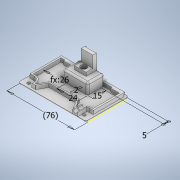
# Autodesk Inventor part: Deckel
Saved by Autodesk Inventor 2020.3 (Build 243373000, 373)
## iProperties
Created: 2020-09-26
Part Number: Deckel
Material: Generisch
Document SubType Name: Modeling
Designer: hpcwoess
Density: 1 g/cm^3
Appearance: Vorgabe
Author: hpcwoess
Autodesk Inventor part; units mm, degrees
ref_plane "YZ Plane" through (0, 0, 0) normal (1, 0, 0) x (0, 1, 0)
ref_plane "XY Plane" through (0, 0, 0) normal (0, 0, 1) x (1, 0, 0)
ref_plane "Arbeitsebene1" through (-34.5, -94, 30.7) normal (0, 1, 0) x (-1, 0, 0)
sketch "Skizze1" plane through (-34.5, -94, 30.7) normal (0, 1, 0) x (-1, 0, 0)
  circle A0 centre (-5, 5) radius 1.75 projected
  circle A1 centre (-67, 5) radius 1.75 projected
  arc A2 (-54.3246, 3.4866) -> (-54.0238, 3.1454) centre (-53.4437, 3.96) ccw projected
  line L0 (-54.3246, 3.4866) -> (-56.467, 7.4734) projected
  arc A3 (-56.467, 7.4734) -> (-57.3479, 8) centre (-57.3479, 7) ccw projected
  line L1 (-10, 8) -> (-14.6521, 8) projected
  arc A4 (-67, 0) -> (-65.2, 0.3352) centre (-67, 5) ccw projected
  line L2 (-67, 0) -> (-72, 0) projected
  line L3 (-72, 0) -> (-72, -34.5) projected
  line L4 (-62, -34.5) -> (-72, -34.5) projected
  line L5 (-62, -36) -> (-62, -34.5) projected
  line L6 (-62, -36) -> (-26, -36) projected
  line L7 (-26, -36) -> (-26, -34.5) projected
  line L8 (-9, -34.5) -> (-26, -34.5) projected
  line L9 (-9, -36) -> (-9, -34.5) projected
  line L10 (-9, -36) -> (-1, -36) projected
  arc A5 (-1, -36) -> (0, -35) centre (-1, -35) ccw projected
  line L11 (0, -35) -> (0, 0) projected
  line L12 (0, 0) -> (-5, 0) projected
  arc A6 (-10, 5) -> (-5, 0) centre (-5, 5) ccw projected
  line L13 (-10, 5) -> (-10, 8) projected
  arc A7 (-14.6521, 8) -> (-15.533, 7.4734) centre (-14.6521, 7) ccw projected
  line L14 (-15.533, 7.4734) -> (-20.4626, -1.7) projected
  line L15 (-24.2, -1.7) -> (-20.4626, -1.7) projected
  arc A8 (-24.2, -1.7) -> (-24.2487, -0.7) centre (-34.5, -1.7) ccw projected
  line L16 (-24.2487, -0.7) -> (-22.25, -0.7) projected
  line L17 (-22.25, 8) -> (-22.25, -0.7) projected
  line L18 (-22.25, 8) -> (-49.75, 8) projected
  line L19 (-49.75, -0.7) -> (-49.75, 8) projected
  line L20 (-49.75, -0.7) -> (-47, -0.7) projected
  line L21 (-47, -1.7) -> (-47, -0.7) projected
  line L22 (-50.4728, -1.7) -> (-47, -1.7) projected
  arc A9 (-50.4728, -1.7) -> (-54.0238, 3.1454) centre (-59.5709, -4.6437) ccw projected
  arc A10 (-74, -36) -> (-72, -38) centre (-72, -36) ccw projected
  line L23 (-74, -36) -> (-74, 8) projected
  arc A11 (-72, 10) -> (-74, 8) centre (-72, 8) ccw projected
  line L24 (-58.8, 10) -> (0, 10) projected
  arc A12 (2, 8) -> (0, 10) centre (0, 8) ccw projected
  line L25 (2, 8) -> (2, -36) projected
  arc A13 (0, -38) -> (2, -36) centre (0, -36) ccw projected
  line L26 (0, -38) -> (-72, -38) projected
  line L27 (-26.4, -35.6) -> (-61.6, -35.6)
  line L28 (-61.6, -35.6) -> (-61.6, -34.1)
  line L29 (-61.6, -34.1) -> (-71.6, -34.1)
  line L30 (-71.6, -34.1) -> (-71.6, -0.4)
  line L31 (-71.6, -0.4) -> (-67, -0.4)
  arc A14 (-67, -0.4) -> (-61.624, 4.4915) centre (-67, 5) ccw
  line L32 (-61.624, 4.4915) -> (-61.624, 7.6)
  line L33 (-61.624, 7.6) -> (-57.3479, 7.6)
  arc A15 (-56.8193, 7.284) -> (-57.3479, 7.6) centre (-57.3479, 7) ccw
  line L34 (-56.8193, 7.284) -> (-54.6769, 3.2973)
  arc A16 (-54.6769, 3.2973) -> (-54.2558, 2.8196) centre (-53.4437, 3.96) ccw
  arc A17 (-50.7686, -2.1) -> (-54.2558, 2.8196) centre (-59.5709, -4.6437) ccw
  line L35 (-50.7686, -2.1) -> (-46.6, -2.1)
  line L36 (-46.6, -2.1) -> (-46.6, -0.3)
  line L37 (-46.6, -0.3) -> (-49.35, -0.3)
  line L38 (-49.35, -0.3) -> (-49.35, 7.6)
  line L39 (-49.35, 7.6) -> (-22.65, 7.6)
  line L40 (-22.65, 7.6) -> (-22.65, -0.3)
  line L41 (-22.65, -0.3) -> (-24.6995, -0.3)
  arc A18 (-24.6081, -2.1) -> (-24.6995, -0.3) centre (-34.5, -1.7) ccw
  line L42 (-24.6081, -2.1) -> (-20.2235, -2.1)
  line L43 (-20.2235, -2.1) -> (-15.1807, 7.284)
  arc A19 (-14.6521, 7.6) -> (-15.1807, 7.284) centre (-14.6521, 7) ccw
  line L44 (-14.6521, 7.6) -> (-10.4, 7.6)
  line L45 (-10.4, 7.6) -> (-10.4, 5)
  arc A20 (-10.4, 5) -> (-5, -0.4) centre (-5, 5) ccw
  line L46 (-5, -0.4) -> (-0.4, -0.4)
  line L47 (-0.4, -0.4) -> (-0.4, -35)
  arc A21 (-1, -35.6) -> (-0.4, -35) centre (-1, -35) ccw
  line L48 (-1, -35.6) -> (-8.6, -35.6)
  line L49 (-8.6, -35.6) -> (-8.6, -34.1)
  line L50 (-8.6, -34.1) -> (-26.4, -34.1)
  line L51 (-26.4, -34.1) -> (-26.4, -35.6)
  line L52 (-59.6, -33.6) -> (-28.4, -33.6)
  line L53 (-28.4, -33.6) -> (-28.4, -32.1)
  line L54 (-28.4, -32.1) -> (-6.6, -32.1)
  line L55 (-6.6, -32.1) -> (-6.6, -33.6)
  line L56 (-6.6, -33.6) -> (-2.4, -33.6)
  line L57 (-2.4, -33.6) -> (-2.4, -2.4)
  line L58 (-2.4, -2.4) -> (-5, -2.4)
  arc A22 (-12.4, 5) -> (-5, -2.4) centre (-5, 5) ccw
  line L59 (-12.4, 5) -> (-12.4, 5.6)
  line L60 (-12.4, 5.6) -> (-13.8151, 5.6)
  line L61 (-13.8151, 5.6) -> (-19.0277, -4.1)
  line L62 (-19.0277, -4.1) -> (-26.9734, -4.1)
  arc A23 (-26.9734, -4.1) -> (-27.3691, 1.7) centre (-34.5, -1.7) ccw
  line L63 (-27.3691, 1.7) -> (-24.65, 1.7)
  line L64 (-24.65, 1.7) -> (-24.65, 5.6)
  line L65 (-24.65, 5.6) -> (-47.35, 5.6)
  line L66 (-47.35, 5.6) -> (-47.35, 1.7)
  line L67 (-47.35, 1.7) -> (-44.6, 1.7)
  line L68 (-44.6, 1.7) -> (-44.6, -4.1)
  line L69 (-44.6, -4.1) -> (-52.4291, -4.1)
  arc A24 (-52.4291, -4.1) -> (-55.416, 1.1905) centre (-59.5709, -4.6437) ccw
  arc A25 (-56.4387, 2.3505) -> (-55.416, 1.1905) centre (-53.4437, 3.96) ccw
  line L70 (-56.4387, 2.3505) -> (-58.1849, 5.6)
  line L71 (-58.1849, 5.6) -> (-59.624, 5.6)
  line L72 (-59.624, 5.6) -> (-59.624, 4.4046)
  arc A26 (-67, -2.4) -> (-59.624, 4.4046) centre (-67, 5) ccw
  line L73 (-67, -2.4) -> (-69.6, -2.4)
  line L74 (-69.6, -2.4) -> (-69.6, -32.1)
  line L75 (-69.6, -32.1) -> (-59.6, -32.1)
  line L76 (-59.6, -32.1) -> (-59.6, -33.6)
  line L77 (-65.2, 10) -> (-65.2, 0.3352) projected
  line L78 (-57.3479, 8) -> (-58.8, 8) projected
  line L79 (-58.8, 8) -> (-58.8, 10) projected
  line L80 (-72, 10) -> (-65.2, 10) projected
  line L81 (-58.8, 10) -> (-65.2, 10)
  line L82 (-58.8, 8) -> (-61.8, 8)
  line L83 (-61.8, 8) -> (-61.8, 4.5)
  point P0 (-34.5, -30.7)
  dimension "d0" = 0.4
  dimension "d1" = 2
  constraints: 106 end point, 26 point on circle, 13 centre point, 2 horizontal, 1 perpendicular, 57 other
  measures "d0" distance between parallel lines of L6 L27
  measures "d1" distance between parallel lines of L27 L52
extrude "Extrusion1" add sketch "Skizze1" against normal blind 2 contours L0 A3 L78 L79 L24 A12 L25 A13 L26 A10 L23 A11 L80 L77 A4 L2 L3 L4 L5 L6 L7 L8 L9 L10 A5 L11 L12 A6 L13 L1 A7 L14 L15 A8 L16 L17 L18 L19 L20 L21 L22 A9 A2 | A2 A9 L22 L21 L20 L19 L18 L17 L16 A8 L15 L14 A7 L1 L13 A6 L12 L11 A5 L10 L9 L8 L7 L6 L5 L4 L3 L2 A4 L77 L81 L79 L78 A3 L0 | L27 L28 L29 L30 L31 A14 L32 L33 A15 L34 A16 A17 L35 L36 L37 L38 L39 L40 L41 A18 L42 L43 A19 L44 L45 A20 L46 L47 A21 L48 L49 L50 L51 | L76 L75 L74 L73 A26 L72 L71 L70 A25 A24 L69 L68 L67 L66 L65 L64 L63 A23 L62 L61 L60 L59 A22 L58 L57 L56 L55 L54 L53 L52
sketch "Skizze4" plane through (-34.5, -94, 30.7) normal (0, 1, 0) x (-1, 0, 0)
  circle A0 centre (-5, 5) radius 1.75
  circle A1 centre (-67, 5) radius 1.75
  arc A2 (-54.3246, 3.4866) -> (-54.0238, 3.1454) centre (-53.4437, 3.96) ccw
  line L0 (-54.3246, 3.4866) -> (-56.467, 7.4734)
  arc A3 (-56.467, 7.4734) -> (-57.3479, 8) centre (-57.3479, 7) ccw
  line L1 (-57.3479, 8) -> (-62.024, 8)
  line L2 (-62.024, 8) -> (-62.024, 4.5108)
  arc A4 (-67, 0) -> (-62.024, 4.5108) centre (-67, 5) ccw
  line L3 (-67, 0) -> (-72, 0)
  line L4 (-72, 0) -> (-72, -34.5)
  line L5 (-62, -34.5) -> (-72, -34.5)
  line L6 (-62, -36) -> (-62, -34.5)
  line L7 (-62, -36) -> (-26, -36)
  line L8 (-26, -36) -> (-26, -34.5)
  line L9 (-9, -34.5) -> (-26, -34.5)
  line L10 (-9, -36) -> (-9, -34.5)
  line L11 (-9, -36) -> (-1, -36)
  arc A5 (-1, -36) -> (0, -35) centre (-1, -35) ccw
  line L12 (0, -35) -> (0, 0)
  line L13 (0, 0) -> (-5, 0)
  arc A6 (-10, 5) -> (-5, 0) centre (-5, 5) ccw
  line L14 (-10, 5) -> (-10, 8)
  line L15 (-10, 8) -> (-14.6521, 8)
  arc A7 (-14.6521, 8) -> (-15.533, 7.4734) centre (-14.6521, 7) ccw
  line L16 (-15.533, 7.4734) -> (-20.4626, -1.7)
  line L17 (-24.2, -1.7) -> (-20.4626, -1.7)
  arc A8 (-24.2, -1.7) -> (-24.2487, -0.7) centre (-34.5, -1.7) ccw
  line L18 (-24.2487, -0.7) -> (-22.25, -0.7)
  line L19 (-22.25, 8) -> (-22.25, -0.7)
  line L20 (-22.25, 8) -> (-49.75, 8)
  line L21 (-49.75, -0.7) -> (-49.75, 8)
  line L22 (-49.75, -0.7) -> (-47, -0.7)
  line L23 (-47, -1.7) -> (-47, -0.7)
  line L24 (-50.4728, -1.7) -> (-47, -1.7)
  arc A9 (-50.4728, -1.7) -> (-54.0238, 3.1454) centre (-59.5709, -4.6437) ccw
  arc A10 (-74, -36) -> (-72, -38) centre (-72, -36) ccw
  line L25 (-74, -36) -> (-74, 8)
  arc A11 (-72, 10) -> (-74, 8) centre (-72, 8) ccw
  line L26 (-72, 10) -> (0, 10)
  arc A12 (2, 8) -> (0, 10) centre (0, 8) ccw
  line L27 (2, 8) -> (2, -36)
  arc A13 (0, -38) -> (2, -36) centre (0, -36) ccw
  line L28 (0, -38) -> (-72, -38)
  line L29 (-26.4, -35.6) -> (-61.6, -35.6)
  line L30 (-61.6, -35.6) -> (-61.6, -34.1)
  line L31 (-61.6, -34.1) -> (-71.6, -34.1)
  line L32 (-71.6, -34.1) -> (-71.6, -0.4)
  line L33 (-71.6, -0.4) -> (-67, -0.4)
  arc A14 (-67, -0.4) -> (-61.624, 4.4915) centre (-67, 5) ccw
  line L34 (-61.624, 4.4915) -> (-61.624, 7.6)
  line L35 (-61.624, 7.6) -> (-57.3479, 7.6)
  arc A15 (-56.8193, 7.284) -> (-57.3479, 7.6) centre (-57.3479, 7) ccw
  line L36 (-56.8193, 7.284) -> (-54.6769, 3.2973)
  arc A16 (-54.6769, 3.2973) -> (-54.2558, 2.8196) centre (-53.4437, 3.96) ccw
  arc A17 (-50.7686, -2.1) -> (-54.2558, 2.8196) centre (-59.5709, -4.6437) ccw
  line L37 (-50.7686, -2.1) -> (-20.2235, -2.1)
  line L38 (-46.6, -0.3) -> (-49.35, -0.3)
  line L39 (-49.35, -0.3) -> (-49.35, 7.6)
  line L40 (-49.35, 7.6) -> (-22.65, 7.6)
  line L41 (-22.65, 7.6) -> (-22.65, -0.3)
  line L42 (-22.65, -0.3) -> (-24.6995, -0.3)
  line L43 (-24.6081, -2.1) -> (-20.2235, -2.1)
  line L44 (-20.2235, -2.1) -> (-15.1807, 7.284)
  arc A18 (-14.6521, 7.6) -> (-15.1807, 7.284) centre (-14.6521, 7) ccw
  line L45 (-14.6521, 7.6) -> (-10.4, 7.6)
  line L46 (-10.4, 7.6) -> (-10.4, 5)
  arc A19 (-10.4, 5) -> (-5, -0.4) centre (-5, 5) ccw
  line L47 (-5, -0.4) -> (-0.4, -0.4)
  line L48 (-0.4, -0.4) -> (-0.4, -35)
  arc A20 (-1, -35.6) -> (-0.4, -35) centre (-1, -35) ccw
  line L49 (-1, -35.6) -> (-8.6, -35.6)
  line L50 (-8.6, -35.6) -> (-8.6, -34.1)
  line L51 (-8.6, -34.1) -> (-26.4, -34.1)
  line L52 (-26.4, -34.1) -> (-26.4, -35.6)
  line L53 (-59.6, -33.6) -> (-28.4, -33.6)
  line L54 (-28.4, -33.6) -> (-28.4, -32.1)
  line L55 (-28.4, -32.1) -> (-6.6, -32.1)
  line L56 (-6.6, -32.1) -> (-6.6, -33.6)
  line L57 (-6.6, -33.6) -> (-2.4, -33.6)
  line L58 (-2.4, -33.6) -> (-2.4, -2.4)
  line L59 (-2.4, -2.4) -> (-5, -2.4)
  arc A21 (-12.4, 5) -> (-5, -2.4) centre (-5, 5) ccw
  line L60 (-12.4, 5) -> (-12.4, 5.6)
  line L61 (-12.4, 5.6) -> (-13.8151, 5.6)
  line L62 (-13.8151, 5.6) -> (-19.0277, -4.1)
  line L63 (-19.0277, -4.1) -> (-26.9734, -4.1)
  line L64 (-27.3691, 1.7) -> (-24.65, 1.7)
  line L65 (-24.65, 1.7) -> (-24.65, 5.6)
  line L66 (-24.65, 5.6) -> (-47.35, 5.6)
  line L67 (-47.35, 5.6) -> (-47.35, 1.7)
  line L68 (-47.35, 1.7) -> (-44.6, 1.7)
  line L69 (-19.0277, -4.1) -> (-52.4291, -4.1)
  arc A22 (-52.4291, -4.1) -> (-55.416, 1.1905) centre (-59.5709, -4.6437) ccw
  arc A23 (-56.4387, 2.3505) -> (-55.416, 1.1905) centre (-53.4437, 3.96) ccw
  line L70 (-56.4387, 2.3505) -> (-58.1849, 5.6)
  line L71 (-58.1849, 5.6) -> (-59.624, 5.6)
  line L72 (-59.624, 5.6) -> (-59.624, 4.4046)
  arc A24 (-67, -2.4) -> (-59.624, 4.4046) centre (-67, 5) ccw
  line L73 (-67, -2.4) -> (-69.6, -2.4)
  line L74 (-69.6, -2.4) -> (-69.6, -32.1)
  line L75 (-69.6, -32.1) -> (-59.6, -32.1)
  line L76 (-59.6, -32.1) -> (-59.6, -33.6)
  point P0 (-34.5, -30.7)
  point P1 (-34.5, -30.7)
  point P2 (-26.9734, -4.1)
  dimension "d4" = 0.4
  dimension "d5" = 2
  constraints: 154 end point, 46 point on circle, 25 centre point, 51 other
  measures "d4" distance between parallel lines of L7 L29
  measures "d5" distance between parallel lines of L29 L53
extrude "Extrusion2" add sketch "Skizze4" along normal blind 4 contours L29 L30 L31 L32 L33 A14 L34 L35 A15 L36 A16 A17 L37 L44 A18 L45 L46 A19 L47 L48 A20 L49 L50 L51 L52
sketch "Skizze5" plane through (-34.5, -96, 30.7) normal (0, -1, 0) x (1, 0, 0)
  line L0 (24, -18) -> (48, -18)
  line L1 (48, -18) -> (48, -33)
  line L2 (48, -33) -> (24, -33)
  line L3 (24, -33) -> (24, -18)
  line L4 (-2, 8) -> (-2, -36) projected
  line L5 (74, -36) -> (74, 8) projected
  line L6 (0, -38) -> (72, -38) projected
  line L7 (50, -16) -> (22, -16)
  line L8 (22, -16) -> (22, -35)
  line L9 (22, -35) -> (50, -35)
  line L10 (50, -35) -> (50, -16)
  point P0 (34.5, -30.7)
  dimension "d8" = 24
  dimension "d9" = 15
  dimension "d10" = 26
  dimension "d11" = 76
  dimension "d12" = 5
  dimension "d13" = 2
  constraints: 16 end point, 4 parallel, 2 perpendicular, 1 horizontal, 3 other
  measures "d8" distance of L0.start L0.end
  measures "d9" distance of L0.end L1.end
  measures "d10" distance between parallel lines of L4 L3
  measures "d11" distance between parallel lines of L5 L4
  measures "d12" distance between parallel lines of L2 L6
  measures "d13" distance between parallel lines of L0 L7
extrude "Extrusion3" add sketch "Skizze5" against normal blind 14 contours L0 L1 L2 L3 | L10 L9 L8 L7
extrude "Extrusion4" cut sketch "Skizze5" against normal blind 12 contours L0 L1 L2 L3
sketch "Skizze6" plane through (-34.5, -84, 30.7) normal (0, -1, 0) x (1, 0, 0)
  circle A0 centre (36, -25.5) radius 3.25
  line L0 (48, -18) -> (48, -33) projected
  line L1 (24, -18) -> (48, -18) projected
  line L2 (29.5, -21.75) -> (42.5, -21.75)
  line L3 (42.5, -21.75) -> (42.5, -29.25)
  line L4 (42.5, -29.25) -> (29.5, -29.25)
  line L5 (29.5, -29.25) -> (29.5, -21.75)
  line L6 (50, -35) -> (22, -35) projected
  line L7 (29.5, -29.25) -> (42.5, -29.25)
  line L8 (42.5, -29.25) -> (42.5, -35)
  line L9 (42.5, -35) -> (29.5, -35)
  line L10 (29.5, -35) -> (29.5, -29.25)
  point P0 (34.5, -30.7)
  dimension "d18" = 6.5
  dimension "d19" = 12
  dimension "d20" = 7.5
  dimension "d25" = 7.5
  dimension "d26" = 3.75
  dimension "d27" = 13
  dimension "d28" = 6.5
  constraints: 16 end point, 4 parallel, 2 horizontal, 2 perpendicular, 2 point on line, 1 centre point
  measures "d18" diameter of A0
  measures "d19" distance from line of A0.centre L0
  measures "d20" distance from line of L1 A0.centre
  measures "d25" distance between parallel lines of L2 L4
  measures "d26" distance from line of L4 A0.centre
  measures "d27" distance of L2.start L2.end
  measures "d28" distance from line of L3 A0.centre
sketch "Skizze7" plane through (37.1, -94, -3.4) normal (1, 0, 0) x (0, 0, -1)
  line L0 (1.5, 4) -> (0.9, 4) projected
  line L1 (3.9, 0) -> (3.9, -2) projected
  line L2 (1.5, 4) -> (3.9, 4)
  line L3 (3.9, 4) -> (3.9, 0)
  line L4 (3.9, 0) -> (1.5, 0)
  line L5 (1.5, 0) -> (1.5, 4)
  line L6 (3.9, 0) -> (2.2, 0)
  line L7 (2.2, 0) -> (2.2, 2.2)
  line L8 (2.2, 2.2) -> (3.9, 2.2)
  line L9 (3.9, 2.2) -> (3.9, 0)
  line L10 (0, 0) -> (0, 4) projected
  line L11 (1.5, 4) -> (0, 4)
  line L12 (0, 4) -> (0, 0)
  line L13 (0, 0) -> (1.5, 0)
  line L14 (1.5, 0) -> (1.5, 4)
  point P0 (-3.4, 94)
  point P1 (2.2, 0)
  point P2 (3.9, 2.2)
  point P3 (1.5, 0)
  dimension "d21" = 1.7
  dimension "d22" = 2.2
  constraints: 24 end point, 6 parallel, 3 horizontal, 3 perpendicular
  measures "d21" distance of L7.end L8.end
  measures "d22" distance of L6.end L7.end
extrude "Extrusion5" add sketch "Skizze7" against normal up to surface (71.2 mm away) contours L5 L13 L10 L11 L0 | L2 L3 L8 L7 L4 L5
sketch "Skizze8" plane through (-34.5, -96, 30.7) normal (0, -1, 0) x (1, 0, 0)
  point P0 (34.5, -30.7)
extrude "Extrusion6" add sketch "Skizze6" against normal blind 6 contours L2 L3 L4 L5
sketch "Skizze9" plane through (-34.5, -84, 30.7) normal (0, -1, 0) x (1, 0, 0)
  circle A0 centre (36, -25.5) radius 3.25
  line L0 (48, -18) -> (48, -33)
  line L1 (24, -18) -> (48, -18)
  line L2 (29.5, -21.75) -> (42.5, -21.75)
  line L3 (42.5, -21.75) -> (42.5, -29.25)
  line L4 (42.5, -29.25) -> (29.5, -29.25)
  line L5 (29.5, -29.25) -> (29.5, -21.75)
  line L6 (50, -35) -> (22, -35)
  line L7 (29.5, -29.25) -> (42.5, -29.25)
  line L8 (42.5, -29.25) -> (42.5, -35)
  line L9 (42.5, -35) -> (29.5, -35)
  line L10 (29.5, -35) -> (29.5, -29.25)
  point P0 (34.5, -30.7)
  point P1 (34.5, -30.7)
  dimension "d31" = 6.5
  dimension "d32" = 12
  dimension "d33" = 7.5
  dimension "d34" = 7.5
  dimension "d35" = 3.75
  dimension "d36" = 13
  dimension "d37" = 6.5
  constraints: 22 end point, 4 parallel, 2 horizontal, 2 perpendicular, 2 point on line, 1 centre point
  measures "d31" diameter of A0
  measures "d32" distance from line of A0.centre L0
  measures "d33" distance from line of L1 A0.centre
  measures "d34" distance between parallel lines of L2 L4
  measures "d35" distance from line of L4 A0.centre
  measures "d36" distance of L2.start L2.end
  measures "d37" distance from line of L3 A0.centre
extrude "Extrusion7" add sketch "Skizze9" against normal blind 19 contours L4 L8 L6 L10
sketch "Skizze10" plane through (-34.5, -78, 30.7) normal (0, 1, 0) x (1, 0, 0)
  line L0 (29.5, 21.75) -> (42.5, 21.75) projected
  line L1 (42.5, 21.75) -> (42.5, 29.25) projected
  line L2 (42.5, 29.25) -> (29.5, 29.25) projected
  line L3 (29.5, 29.25) -> (29.5, 21.75) projected
  circle A0 centre (36, 25.5) radius 3.25 projected
  point P0 (34.5, 30.7)
extrude "Extrusion8" cut sketch "Skizze10" against normal blind 10 contours A0
fillet "Rundung1" radius 2 20 edges at (1.5, -96, 12.7) (13.5, -96, 5.2) (1.5, -96, -2.3) (-10.5, -96, 5.2) (1.5, -82, 14.7) (15.5, -82, 5.2) (1.5, -84, -2.3) (-10.5, -84, 5.2) (1.5, -84, 12.7) (13.5, -84, 5.2) (-12.5, -82, 5.2) (15.5, -88, 14.7) (-12.5, -88, 14.7) (1.5, -65, -4.3) (8, -73.5, -4.3) (-5, -73.5, -4.3) (11.75, -82, -4.3) (-8.75, -82, -4.3) (15.5, -86, -4.3) (-12.5, -86, -4.3)
fillet "Rundung2" radius 2 7 edges at (-35.9142, -96, 40.1142) (-36.5, -96, 16.7) (-35.9142, -96, -6.7142) (1.5, -96, -7.3) (38.9142, -96, -6.7142) (39.5, -96, 16.7) (38.9142, -96, 40.1142)
sketch "Skizze11" plane through (-34.5, -84, 30.7) normal (0, -1, 0) x (1, 0, 0)
  line L0 (27.3428, -21.9377) -> (49.5374, -21.9377) construction
  line L1 (49.5374, -21.9377) -> (49.5374, -30.3697) construction
  line L2 (49.5374, -30.3697) -> (27.3428, -30.3697) construction
  line L3 (27.3428, -30.3697) -> (27.3428, -21.9377) construction
  line L4 (30.4911, -29.0852) -> (27.7796, -29.0852)
  line L5 (27.7796, -29.0852) -> (27.7796, -28.3705)
  line L6 (27.7796, -28.3705) -> (28.6702, -28.3705)
  line L7 (28.6702, -28.3705) -> (28.6702, -22.8)
  line L8 (28.6702, -22.8) -> (27.7796, -22.8)
  line L9 (27.7796, -22.8) -> (27.7796, -22.0852)
  line L10 (27.7796, -22.0852) -> (30.4911, -22.0852)
  line L11 (30.4911, -22.0852) -> (30.4911, -22.8)
  line L12 (30.4911, -22.8) -> (29.6005, -22.8)
  line L13 (29.6005, -22.8) -> (29.6005, -28.3705)
  line L14 (29.6005, -28.3705) -> (30.4911, -28.3705)
  line L15 (30.4911, -28.3705) -> (30.4911, -29.0852)
  spline S0 degree 2 poles (45.6143, -22.8851) (46.0114, -23.3502) (46.4538, -24.7116) (46.4538, -25.5852) knots 0 0 0 1 2 2 2
  spline S1 degree 2 poles (46.4538, -25.5852) (46.4538, -26.4361) (46.0227, -27.8145) (45.6143, -28.2797) knots 0 0 0 1 2 2 2
  spline S2 degree 2 poles (45.6143, -28.2797) (45.1832, -28.7675) (44.043, -29.2327) (43.3566, -29.2327) knots 0 0 0 1 2 2 2
  spline S3 degree 2 poles (43.3566, -29.2327) (42.6475, -29.2327) (41.513, -28.7505) (41.0989, -28.2797) knots 0 0 0 1 2 2 2
  spline S4 degree 2 poles (41.0989, -28.2797) (40.6961, -27.8145) (40.265, -26.4474) (40.265, -25.5852) knots 0 0 0 1 2 2 2
  spline S5 degree 2 poles (40.265, -25.5852) (40.265, -24.706) (40.7018, -23.3672) (41.1046, -22.8851) knots 0 0 0 1 2 2 2
  spline S6 degree 2 poles (41.1046, -22.8851) (41.513, -22.4199) (42.6532, -21.9377) (43.3566, -21.9377) knots 0 0 0 1 2 2 2
  spline S7 degree 2 poles (43.3566, -21.9377) (44.0714, -21.9377) (45.2172, -22.4369) (45.6143, -22.8851) knots 0 0 0 1 2 2 2
  spline S8 degree 2 poles (45.4838, -25.5852) (45.4838, -24.8932) (45.1832, -23.821) (44.9109, -23.4693) knots 0 0 0 1 2 2 2
  spline S9 degree 2 poles (44.9109, -23.4693) (44.6329, -23.1063) (43.8501, -22.7432) (43.3623, -22.7432) knots 0 0 0 1 2 2 2
  spline S10 degree 2 poles (43.3623, -22.7432) (42.8574, -22.7432) (42.0973, -23.0949) (41.808, -23.4693) knots 0 0 0 1 2 2 2
  spline S11 degree 2 poles (41.808, -23.4693) (41.53, -23.8267) (41.235, -24.9045) (41.235, -25.5852) knots 0 0 0 1 2 2 2
  spline S12 degree 2 poles (41.235, -25.5852) (41.235, -26.9637) (42.3923, -28.4272) (43.3623, -28.4272) knots 0 0 0 1 2 2 2
  spline S13 degree 2 poles (43.3623, -28.4272) (44.3323, -28.4272) (45.4838, -26.9637) (45.4838, -25.5852) knots 0 0 0 1 2 2 2
  point P0 (34.5, -30.7)
  constraints: 2 other
extrude "Extrusion9" cut sketch "Skizze11" against normal mid plane 1
chamfer "Fase1" distance 0.5 distance2 4 1 edges at (0.9961, -90, 28.6) measured on face at (0.9961, -90, 28.1)
chamfer "Fase2" distance 0.5 distance2 4 6 edges at (16.2005, -90, 28.351) (17.5959, -90, 31.3549) (19.9939, -90, 33.7342) (21.2481, -90, 35.9906) (22.54, -90, 38.215) (24.9859, -90, 38.3) measured on face at (16.6845, -90, 28.2257) measured on face at (21.6886, -90, 35.754) measured on face at (24.9859, -90, 37.8) measured on face at (18.0038, -90, 31.0658) measured on face at (22.7965, -90, 37.7858) measured on face at (20.369, -90, 33.4035)
chamfer "Fase3" distance 0.5 distance2 4 2 edges at (28.8658, -90, 31.7059) (34.8, -90, 30.3)
chamfer "Fase4" distance 0.5 distance2 4 1 edges at (27.124, -90, 35.5347) measured on face at (26.624, -90, 35.5347)
chamfer "Fase5" distance 0.5 distance2 4 3 edges at (-16.6636, -90, 33.0421) (-19.54, -90, 38.215) (-21.9739, -90, 38.3) measured on face at (-19.7965, -90, 37.7858) measured on face at (-21.9739, -90, 37.8) measured on face at (-17.104, -90, 32.8054)
chamfer "Fase6" distance 0.5 distance2 4 3 edges at (-25.6816, -90, 31.8816) (-24.1, -90, 36.75) (-31.8, -90, 30.3) measured on face at (-25.3281, -90, 31.5281) measured on face at (-23.6, -90, 36.75) measured on face at (-31.8, -90, 29.8)
sketch "Skizze12" plane through (-34.5, -94, 30.7) normal (0, 1, 0) x (1, 0, 0)
  line L0 (0, -10) -> (59, -10) projected
  line L1 (65, -10) -> (59, -10)
  line L2 (59, -10) -> (59, 0)
  line L3 (59, 0) -> (65, 0)
  line L4 (65, 0) -> (65, -10)
  circle A0 centre (67, -5) radius 1.75 projected
  point P0 (34.5, 30.7)
  point P1 (72, -10)
  dimension "d66" = 6
  dimension "d67" = 10
  dimension "d68" = 2
  constraints: 8 end point, 2 parallel, 1 horizontal, 1 perpendicular, 1 point on line
  measures "d66" distance of L2.end L3.end
  measures "d67" distance of L0.end L2.end
  measures "d68" distance from line of A0.centre L4
extrude "Extrusion10" add sketch "Skizze12" along normal blind 4 contours L1 L2 L3 L4
sketch "Skizze13" plane through (-34.5, -90, 30.7) normal (0, 1, 0) x (1, 0, 0)
  line L0 (65, -10) -> (65, 0) projected
  line L1 (59, -7.1) -> (59, -5.6) projected
  line L2 (59, -10) -> (65, -10) projected
  line L3 (62, -10) -> (62, 0)
  line L4 (65, 0) -> (63.8679, 0) projected
  line L5 (60, 0) -> (60, -10)
  line L6 (64, 0) -> (64, -10)
  line L7 (60, -4.5) -> (60.1, -4.5)
  line L8 (60.1, -4.5) -> (60.1, -5.5)
  line L9 (60.1, -5.5) -> (60, -5.5)
  line L10 (60, -5.5) -> (60, -4.5)
  line L11 (60, 0) -> (62, 0)
  line L12 (61.5447, 0) -> (59, 0) projected
  line L13 (60, -10) -> (62, -10)
  line L14 (60, 0) -> (62, 0)
  line L15 (62, 0) -> (62, 3.925)
  line L16 (62, 3.925) -> (60, 3.925)
  line L17 (60, 3.925) -> (60, 0)
  point P0 (34.5, 30.7)
  point P1 (62, 0)
  dimension "d72" = 2
  dimension "d73" = 2
  dimension "d74" = 0.1
  dimension "d75" = 1
  dimension "d76" = 4.5
  constraints: 26 end point, 4 parallel, 4 point on line, 3 perpendicular, 2 collinear, 2 horizontal, 2 vertical, 1 midpoint
  measures "d72" distance between parallel lines of L5 L3
  measures "d73" distance between parallel lines of L6 L3
  measures "d74" distance of L8.end L9.end
  measures "d75" distance of L7.end L8.end
  measures "d76" distance from line of L8.end L2
revolve "Umdrehung1" cut sketch "Skizze13" angle 360 about axis through (27.5, -90, 40.7) along (0, 0, -1) contours L5 L9 L8 L7 L11 L3 L2 | L11 L17 L16 L15
sketch "Skizze14" plane through (37.1, -94, -5.6) normal (1, 0, 0) x (0, 0, -1)
  line L0 (-2, 0) -> (-2, 2.1901)
  line L1 (-2, 2.1901) -> (-0.3, 2.1901)
  line L2 (-0.3, 2.1901) -> (-0.3, 4)
  line L3 (-0.3, 4) -> (1.7, 4)
  line L4 (1.7, 4) -> (1.7, 0)
  line L5 (1.7, 0) -> (-2.2122, 0)
  line L6 (0, 0) -> (-35.9, 0) projected
  line L7 (-44.3, 0) -> (-0.3, 0) projected
  line L8 (-35.4, 4) -> (1.7, 4) projected
  line L9 (0, 0) -> (0, 2.2) projected
  point P0 (-5.6, 94)
  point P1 (-2, 0)
  dimension "d78" = 2
  dimension "d79" = 2
  constraints: 12 end point, 3 perpendicular, 3 point on line, 1 horizontal, 1 vertical
  measures "d78" distance between parallel lines of L4 L2
  measures "d79" distance between parallel lines of L9 L0
extrude "Extrusion11" cut sketch "Skizze14" against normal through all
equation "\"d10\" = -0.5 * d8 + 0.5 * d11"
equation "\"d19\" = 0.5 * d8"
equation "\"d20\" = 0.5 * d9"
equation "\"d26\" = 0.5 * d25"
equation "\"d28\" = 0.5 * d27"
equation "\"d32\" = 0.5 * d38"
equation "\"d33\" = 0.5 * d39"
equation "\"d35\" = 0.5 * d34"
equation "\"d37\" = 0.5 * d36"
equation "\"d73\" = d72"
equation "\"d79\" = d78"
equation "\"d38\" = 24"
equation "\"d39\" = 15"
